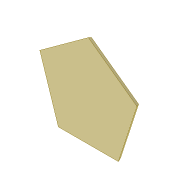
# Autodesk Inventor part: Face
Saved by Autodesk Inventor 2022.2 (Build 262287010, 287A)
## iProperties
Created: 2022-12-30
Part Number: Face
Material: Gold
Document SubType Name: Modeling
Designer: User
Mass: 90.5024 g
Surface Area: 50.8817 cm^2
Volume: 4.68924 cm^3
Density: 19.3 g/cm^3
Appearance: Gold - Metal
Author: User
Autodesk Inventor part; units mm, degrees
ref_plane "YZ Plane" through (0, 0, 0) normal (1, 0, 0) x (0, 1, 0)
ref_plane "XZ Plane" through (0, 0, 0) normal (0, 1, 0) x (-1, 0, 0)
ref_plane "XY Plane" through (0, 0, 0) normal (0, 0, 1) x (1, 0, 0)
sketch "Sketch1" plane through (0, 0, 0) normal (0, 0, 1) x (1, 0, 0)
  line L0 (0, 30.9017) -> (29.3893, 9.5492)
  line L1 (29.3893, 9.5492) -> (18.1636, -25)
  line L2 (18.1636, -25) -> (-18.1636, -25)
  line L3 (-18.1636, -25) -> (-29.3893, 9.5492)
  line L4 (-29.3893, 9.5492) -> (0, 30.9017)
  point P0 (0, 0)
  point P1 (0, 0)
  dimension "d0" = 25
  constraints: 10 end point, 1 coincident, 11 other
  measures "d0" distance from line of L2 point (0, 0)
extrude "Extrusion1" add sketch "Sketch1" along normal blind 2 draft 22
body "Solid1"
